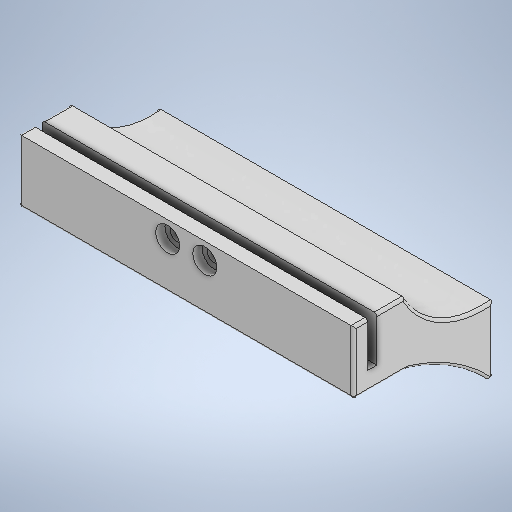
# Autodesk Inventor part: intake wedge
Saved by Autodesk Inventor 2025.1 (Build 291241020, 241B)
## iProperties
Created: 2025-01-10
Part Number: intake wedge
Material: Generic
Document SubType Name: Modeling
Designer: Hunter Mathis
Density: 1 g/cm^3
Appearance: Default
Author: Hunter Mathis
Autodesk Inventor part; units mm, degrees
ref_plane "YZ Plane" through (0, 0, 0) normal (1, 0, 0) x (0, 1, 0)
ref_plane "XZ Plane" through (0, 0, 0) normal (0, 1, 0) x (-1, 0, 0)
ref_plane "XY Plane" through (0, 0, 0) normal (0, 0, 1) x (1, 0, 0)
sketch "Sketch1" plane through (0, 0, 0) normal (0, 0, 1) x (1, 0, 0)
  line L0 (-25.4, 12.7) -> (25.4, 12.7)
  line L1 (25.4, 12.7) -> (25.4, -12.7)
  line L2 (25.4, -12.7) -> (-25.4, -12.7)
  line L3 (-25.4, -12.7) -> (-25.4, 12.7)
  line L4 (-25.4, 12.7) -> (25.4, -12.7) construction
  line L5 (25.4, 12.7) -> (-25.4, -12.7) construction
  point P0 (0, 0)
  dimension "d0" = 50.8
  dimension "d1" = 25.4
  constraints: 12 end point, 2 midpoint, 2 parallel, 1 horizontal, 1 perpendicular
  measures "d0" distance of L1.end L2.end
  measures "d1" distance of L0.end L1.end
extrude "Extrusion1" add sketch "Sketch1" along normal blind 6.35
sketch "Sketch2" plane through (0, 0, 6.35) normal (0, 0, 1) x (1, 0, 0)
  line L0 (-25.4, -12.7) -> (25.4, -12.7) projected
  line L1 (-25.4, -12.7) -> (0, -12.7)
  line L2 (25.4, -12.7) -> (0, -12.7)
  line L3 (25.4, -12.7) -> (12.7, -12.7)
  line L4 (25.4, -12.7) -> (19.05, -12.7)
  line L5 (-25.4, -12.7) -> (-6.35, -12.7)
  line L6 (-6.35, -12.7) -> (6.35, -12.7)
  line L7 (6.35, -12.7) -> (6.35, -4.445)
  line L8 (-6.35, -12.7) -> (-6.35, -4.445)
  line L9 (-6.35, -4.445) -> (-6.35, 12.7)
  line L10 (25.4, 12.7) -> (-25.4, 12.7) projected
  line L11 (-6.35, 12.7) -> (-6.35, 3.175)
  line L12 (6.35, -4.445) -> (6.35, 12.7)
  line L13 (6.35, 12.7) -> (6.35, 3.175)
  circle A0 centre (-6.35, 3.175) radius 2.3241
  circle A1 centre (-6.35, 3.175) radius 4.1275
  circle A2 centre (6.35, 3.175) radius 2.3241
  circle A3 centre (6.35, 3.175) radius 4.1275
  point P0 (0, 0)
  dimension "d33" = 12.7
  dimension "d43" = 9.525
  dimension "d44" = 9.525
  dimension "d45" = 4.6482
  dimension "d46" = 8.255
  dimension "d47" = 4.6482
  dimension "d48" = 8.255
  constraints: 24 end point, 6 point on line, 4 centre point, 4 coincident, 3 midpoint, 2 vertical, 1 collinear, 1 perpendicular
  measures "d33" distance of L5.end L6.end
  measures "d43" distance of L9.end L11.end
  measures "d44" distance of L12.end L13.end
  measures "d45" diameter of A0
  measures "d46" diameter of A1
  measures "d47" diameter of A2
  measures "d48" diameter of A3
sketch "Sketch5" plane through (0, 0, 6.35) normal (0, 0, 1) x (1, 0, 0)
  line L0 (-25.4, -12.7) -> (25.4, -12.7) projected
  line L1 (-25.4, 12.7) -> (-25.4, -12.7) projected
  line L2 (25.4, -12.7) -> (-25.4, -12.7)
  line L3 (-25.4, -12.7) -> (-25.4, 12.7)
  line L4 (-25.4, 12.7) -> (25.4, 12.7)
  line L5 (25.4, 12.7) -> (25.4, -12.7)
  point P0 (0, 0)
  constraints: 8 end point, 2 parallel, 1 horizontal, 1 perpendicular
extrude "Extrusion6" add sketch "Sketch5" along normal blind 3.175
extrude "Extrusion2" cut sketch "Sketch2" along normal mid plane 12.7 contours A0 L9 | L9 A0 | A2 L12 | L12 A2
extrude "Extrusion3" cut sketch "Sketch2" along normal blind 3.175 contours A1 L9 A0 | L9 A0 A1 | A3 L12 A2 | L12 A2 A3
sketch "Sketch4" plane through (-25.4, 12.7, 0) normal (0, 1, 0) x (1, 0, 0)
  line L0 (0, 0) -> (50.8, 0) projected
  line L1 (50.8, 0) -> (50.8, -6.35) projected
  line L2 (50.8, 0) -> (50.8, -1.5875)
  line L3 (0, -6.35) -> (0, 2.7928) projected
  line L4 (0, -3.175) -> (0, -1.5875)
  line L5 (50.8, -3.175) -> (50.8, -1.5875)
  line L6 (0, -6.35) -> (50.8, -6.35) projected
  line L7 (50.8, -6.35) -> (50.8, 0)
  line L8 (50.8, -6.35) -> (50.8, -3.175)
  line L9 (50.8, 0) -> (50.8, -6.35) projected
  line L10 (50.8, -6.35) -> (50.8, -3.175)
  line L11 (50.8, -6.35) -> (50.8, -4.3087)
  line L12 (50.8, 0) -> (50.8, -1.9355)
  line L13 (50.8, -1.9355) -> (50.8, -3.175)
  line L14 (0, -3.175) -> (0, -1.9355)
  line L15 (50.8, -6.35) -> (50.8, 0)
  line L16 (50.8, 0) -> (50.8, -1.5875)
  line L17 (50.8, -6.35) -> (50.8, -4.7498)
  line L18 (50.8, -4.7498) -> (0, -4.7498)
  line L19 (50.8, -4.7498) -> (50.8, -1.5875)
  line L20 (0, -4.7498) -> (0, -1.9355)
  line L21 (0, 0) -> (0, -6.35) projected
  line L22 (50.8, -4.7498) -> (50.8, -1.9355)
  line L23 (0, -1.9355) -> (0, -4.7498)
  line L24 (50.8, 0) -> (50.8, -1.5875)
  line L25 (50.8, -4.7498) -> (50.8, -1.5875)
  line L26 (50.8, -1.5875) -> (0, -1.5875)
  line L27 (0, -1.5875) -> (0, -4.7498)
  line L28 (50.8, -4.7498) -> (50.8, -1.5875)
  line L29 (0, -4.7498) -> (0, -1.5875)
  point P0 (25.4, 0)
  dimension "d42" = 1.6002
  constraints: 48 end point, 16 collinear, 7 point on line, 3 perpendicular, 1 midpoint
  measures "d42" distance of L1.end L17.end
extrude "Extrusion5" cut sketch "Sketch4" against normal blind 19.05 contours L26 L1 L18 L3
sketch "Sketch6" plane through (-25.4, -12.7, 0) normal (-1, 0, 0) x (0, 0, 1)
  line L0 (0, 0) -> (0, 25.4) projected
  line L1 (9.525, 25.4) -> (9.525, 0) projected
  line L2 (0, 25.4) -> (9.525, 25.4)
  line L3 (9.525, 25.4) -> (9.525, 21.59)
  line L4 (9.525, 21.59) -> (0, 21.59)
  line L5 (0, 21.59) -> (0, 25.4)
  point P0 (0, 12.7)
  point P1 (0, 21.59)
  dimension "d54" = 3.81
  constraints: 8 end point, 2 parallel, 1 horizontal, 1 perpendicular, 1 point on line
  measures "d54" distance between parallel lines of L4 L2
extrude "Extrusion7" cut sketch "Sketch6" against normal through all
sketch "Sketch11" plane through (0, 0, 0) normal (0, 0, -1) x (-1, 0, 0)
  line L0 (-25.4, -12.7) -> (-25.4, 8.89) projected
  line L1 (25.4, -12.7) -> (-25.4, -12.7) projected
  line L2 (25.4, 8.89) -> (25.4, -12.7) projected
  line L3 (25.4, 8.89) -> (-25.4, 8.89) projected
  circle A0 centre (-6.35, 3.175) radius 2.3241 projected
  circle A1 centre (6.35, 3.175) radius 2.3241 projected
  point P0 (0, 0)
extrude "Extrusion11" add sketch "Sketch11" along normal blind 38.1
sketch "Sketch12" plane through (-25.4, -6.35, 1.5875) normal (-1, 0, 0) x (0, 0, 1)
  line L0 (-39.6875, -6.35) -> (-39.6875, 15.24) projected
  line L1 (7.9375, -6.35) -> (-39.6875, -6.35) projected
  line L2 (7.9375, 15.24) -> (7.9375, -6.35) projected
  line L3 (3.1623, 15.24) -> (3.1623, 0) projected
  line L4 (3.1623, 0) -> (0, 0) projected
  line L5 (0, 0) -> (0, 15.24) projected
  line L6 (0, 12.065) -> (-26.9875, 12.065) projected
  line L7 (0, 12.065) -> (0, 15.24) projected
  line L8 (0, 15.24) -> (-26.9875, 15.24) projected
  line L9 (-26.9875, 12.065) -> (-26.9875, 15.24) projected
  line L10 (7.9375, 12.065) -> (7.9375, 15.24) projected
  line L11 (7.9375, 15.24) -> (3.1623, 15.24) projected
  line L12 (3.1623, 15.24) -> (3.1623, 12.065) projected
  line L13 (3.1623, 12.065) -> (7.9375, 12.065) projected
  line L14 (7.9375, 15.24) -> (3.1623, 15.24) projected
  line L15 (0, 15.24) -> (-39.6875, 15.24) projected
  point P0 (-1.5875, 6.35)
extrude "Extrusion12" add sketch "Sketch12" along normal blind 31.75
sketch "Sketch13" plane through (25.4, -6.35, 4.7498) normal (1, 0, 0) x (0, 0, -1)
  line L0 (0, 15.24) -> (-4.7752, 15.24) projected
  line L1 (-4.7752, -6.35) -> (-4.7752, 15.24) projected
  line L2 (42.8498, -6.35) -> (-4.7752, -6.35) projected
  line L3 (42.8498, 15.24) -> (42.8498, -6.35) projected
  line L4 (3.1623, 15.24) -> (42.8498, 15.24) projected
  line L5 (3.1623, 15.24) -> (3.1623, 0) projected
  line L6 (3.1623, 0) -> (0, 0) projected
  line L7 (0, 0) -> (0, 15.24) projected
  point P0 (4.7498, 6.35)
extrude "Extrusion13" add sketch "Sketch13" along normal blind 31.75
sketch "Sketch15" plane through (57.15, -6.35, 4.7498) normal (1, 0, 0) x (0, 0, -1)
  line L0 (42.8498, 15.24) -> (42.8498, -6.35) projected
  line L1 (42.8498, -6.1511) -> (42.8498, 15.24)
  line L2 (42.8498, 15.24) -> (42.8498, 4.5444)
  line L3 (42.8498, 15.24) -> (20.8733, 15.24)
  line L4 (3.1623, 15.24) -> (42.8498, 15.24) projected
  line L5 (42.8498, -6.35) -> (42.8498, 15.24)
  line L6 (42.8498, -6.35) -> (42.8498, 4.5444)
  line L7 (42.8498, -6.35) -> (42.8498, -0.9028)
  line L8 (42.8498, 15.24) -> (3.1623, 15.24) projected
  arc A0 (12.6527, 15.24) -> (42.8498, -3.6264) centre (42.9894, 30.1966) ccw
  line L9 (12.6527, 15.24) -> (42.8498, 15.24)
  line L10 (42.8498, 15.24) -> (42.8498, -3.6264)
  line L11 (42.8498, -0.9028) -> (42.8498, 15.24)
  arc A1 (12.6527, 15.24) -> (42.8498, -0.9028) centre (39.5427, 29.226) ccw
  point P0 (4.7498, 6.35)
  point P1 (12.6527, 15.24)
  point P2 (42.8498, -3.6264)
  point P3 (12.6527, 15.24)
  constraints: 18 end point, 5 collinear, 4 point on circle, 3 midpoint, 2 centre point, 2 point on line, 1 vertical
extrude "Extrusion15" cut sketch "Sketch15" against normal through all contours L0 A1 L4 L3
sketch "Sketch18" plane through (-57.15, -6.35, 1.5875) normal (-1, 0, 0) x (0, 0, 1)
  line L0 (-39.6875, -6.35) -> (-39.6875, 15.24) projected
  line L1 (7.9375, -6.35) -> (-39.6875, -6.35) projected
  line L2 (-39.6875, -6.35) -> (-0.9525, -6.35)
  line L3 (-39.6875, -6.35) -> (-28.2575, -6.35)
  line L4 (-28.2575, -6.35) -> (-39.6875, -25.0714)
  line L5 (-39.6875, -25.0714) -> (-39.6875, -6.35)
  point P0 (-1.5875, 6.35)
  point P1 (-39.6875, -3.6264)
  point P2 (-28.2575, -6.35)
  point P3 (-39.6875, -0.9028)
  dimension "d84" = 11.43
  constraints: 8 end point, 1 collinear, 1 perpendicular, 1 point on line
  measures "d84" distance of L0.start L3.end
extrude "Extrusion18" add sketch "Sketch18" against normal up to surface (114.3 mm away)
sketch "Sketch24" plane through (-57.15, -6.35, 1.5875) normal (-1, 0, 0) x (0, 0, 1)
  line L0 (-28.2575, -6.35) -> (7.9375, -6.35) projected
  line L1 (-39.6875, -25.0714) -> (-28.2575, -6.35) projected
  line L2 (-39.6875, -25.0714) -> (-28.2575, -6.35)
  line L3 (-28.2575, -6.35) -> (-10.16, -6.35)
  arc A0 (-10.16, -6.35) -> (-39.6875, -25.0714) centre (7.7352, -67.2206) ccw
  point P0 (-1.5875, 6.35)
  constraints: 4 end point, 2 point on circle, 1 centre point, 1 collinear, 1 horizontal, 1 midpoint
extrude "Extrusion23" add sketch "Sketch24" against normal up to surface (114.3 mm away)
sketch "Sketch22" plane through (-57.15, -31.4214, -38.1) normal (0, -0.5210893, 0.8535022) x (1, 0, 0)
  line L0 (0, 0) -> (114.3, 0) projected
  arc A0 (70.2213, 0) -> (44.449, 0) centre (57.3352, -13.601) ccw
  line L1 (44.449, 0) -> (70.2213, 0)
  arc A1 (70.2213, 0) -> (44.449, 0) centre (57.3352, -7.1734) ccw
  point P0 (57.15, 46.6717)
  constraints: 4 point on circle, 2 centre point, 2 end point, 2 point on line
extrude "Extrusion21" cut sketch "Sketch22" along normal through all both and the other way through all
ref_plane "Work Plane2" through (57.15, 22.876, -65.1027) normal (0, 0, -1) x (-1, 0, 0)
sketch "Sketch23" plane through (57.15, 22.876, -65.1027) normal (0, 0, -1) x (-1, 0, 0)
  circle A0 centre (63.5, -19.701) radius 2.3241 projected
  line L0 (63.5, -24.5424) -> (59.3072, -22.1217)
  line L1 (59.3072, -22.1217) -> (59.3072, -17.2803)
  line L2 (59.3072, -17.2803) -> (63.5, -14.8596)
  line L3 (63.5, -14.8596) -> (67.6928, -17.2803)
  line L4 (67.6928, -17.2803) -> (67.6928, -22.1217)
  line L5 (67.6928, -22.1217) -> (63.5, -24.5424)
  circle A1 centre (50.8, -19.701) radius 2.3241 projected
  line L6 (50.8, -24.5424) -> (46.6072, -22.1217)
  line L7 (46.6072, -22.1217) -> (46.6072, -17.2803)
  line L8 (46.6072, -17.2803) -> (50.8, -14.8596)
  line L9 (50.8, -14.8596) -> (54.9928, -17.2803)
  line L10 (54.9928, -17.2803) -> (54.9928, -22.1217)
  line L11 (54.9928, -22.1217) -> (50.8, -24.5424)
  point P0 (57.15, -22.876)
  constraints: 24 end point, 2 coincident, 26 other
extrude "Extrusion22" cut sketch "Sketch23" against normal blind 60.96 contours L0 L1 L2 L3 L4 L5 | A1 | L6 L7 L8 L9 L10 L11
fillet "Fillet12" radius 0.889 18 edges at (-57.15, -19.9867, -24.6513) (-57.15, -19.3371, -38.1) (-34.9255, -31.4214, -38.1) (35.1107, -31.4214, -38.1) (57.15, -19.9867, -24.6513) (57.15, -3.854, -20.5035) (57.15, -19.3371, -38.1) (0, -12.7, -8.5725) (-57.15, -12.7, 0.4762) (-57.15, -1.905, 9.525) (0, -12.7, 9.525) (57.15, -1.905, 9.525) (57.15, -12.7, 0.4762) (-57.15, -3.854, -20.5035) (-57.15, 8.89, 7.1374) (-57.15, 8.89, -3.1577) (57.15, 8.89, -3.1577) (57.15, 8.89, 7.1374)
body "Solid1"
